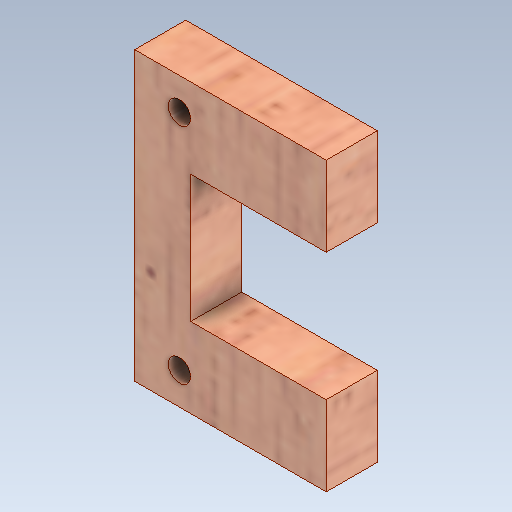
# Autodesk Inventor part: 0005-10-004 Actionare 2 seringa
Saved by Autodesk Inventor 2020 (Build 240168000, 168)
## iProperties
Created: 2020-12-18
Part Number: 0005-10-004 Actionare 2 seringa
Material: Generic
Document SubType Name: Modeling
Designer: Iulian Bors
Density: 1 g/cm^3
Appearance: White Oak - Natural Medium Gloss
Author: Iulian Bors
Subject: 004
Autodesk Inventor part; units mm, degrees
ref_plane "YZ Plane" through (0, 0, 0) normal (1, 0, 0) x (0, 1, 0)
ref_plane "XZ Plane" through (0, 0, 0) normal (0, 1, 0) x (-1, 0, 0)
ref_plane "XY Plane" through (0, 0, 0) normal (0, 0, 1) x (1, 0, 0)
sketch "Sketch1" plane through (0, 0, 0) normal (0, 0, 1) x (1, 0, 0)
  line L0 (-15, 22.5) -> (15, 22.5)
  line L1 (15, 22.5) -> (15, -22.5)
  line L2 (15, -22.5) -> (-15, -22.5)
  line L3 (-15, -22.5) -> (-15, 22.5)
  point P0 (0, 0)
  point P1 (0, 22.5)
  point P2 (-15, 0)
  dimension "d0" = 30
  dimension "d1" = 45
  constraints: 8 end point, 2 midpoint, 2 parallel, 1 horizontal, 1 horizontal alignment, 1 perpendicular, 1 vertical alignment
  measures "d0" distance of L0.start L0.end
  measures "d1" distance of L2.end L0.start
extrude "Extrusion1" add sketch "Sketch1" along normal blind 8
sketch "Sketch3" plane through (0, 0, 0) normal (0, 0, -1) x (-1, 0, 0)
  arc A0 (6.2282, -0.4043) -> (6.2368, 0) centre (-3.25, 0) ccw projected
  line L0 (6.2282, -10) -> (-15, -10)
  line L1 (-15, -10) -> (-15, 10)
  line L2 (-15, 10) -> (6.2282, 10)
  line L3 (6.2282, 10) -> (6.2282, -10)
  line L4 (15, 22.5) -> (15, -22.5) projected
  line L5 (-15, -22.5) -> (-15, 22.5) projected
  point P0 (0, 0)
  point P1 (6.2282, 0)
  point P2 (15, 0)
  dimension "d8" = 0
  dimension "d9" = 20
  constraints: 8 end point, 2 midpoint, 2 parallel, 1 collinear, 1 horizontal, 1 horizontal alignment, 1 perpendicular
  measures "d8" horizontal distance of point (6.228, 0) A0.start
  measures "d9" distance of L2.end L0.start
extrude "Extrusion3" cut sketch "Sketch3" against normal blind 10
sketch "Sketch4" plane through (0, 0, 0) normal (0, 0, -1) x (-1, 0, 0)
  line L0 (-15, -22.5) -> (-15, -10) projected
  line L1 (-15, 10) -> (-15, 22.5) projected
  circle A0 centre (8, 17.5) radius 1.75
  circle A1 centre (8, -17.5) radius 1.75
  line L2 (-15, 22.5) -> (15, 22.5) projected
  line L3 (15, 22.5) -> (15, -22.5) projected
  line L4 (15, -22.5) -> (-15, -22.5) projected
  point P0 (-15, -16.25)
  point P1 (-15, 16.25)
  dimension "d17" = 3.5
  dimension "d18" = 3.5
  dimension "d19" = 5
  dimension "d20" = 7
  dimension "d21" = 5
  dimension "d22" = 35
  constraints: 2 centre point, 2 midpoint, 1 vertical alignment
  measures "d17" diameter of A0
  measures "d18" diameter of A1
  measures "d19" distance from line of A0.centre L2
  measures "d20" distance from line of A0.centre L3
  measures "d21" distance from line of A1.centre L4
  measures "d22" distance of A1.centre A0.centre
extrude "Extrusion4" cut sketch "Sketch4" against normal through all
equation "\"d21\" = d19"
body "Solid1"
